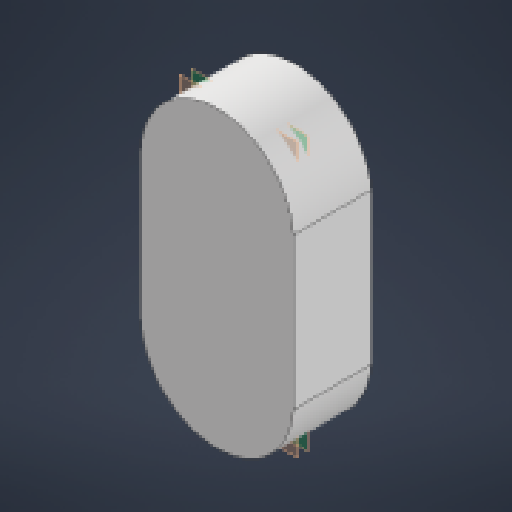
# Autodesk Inventor part: battery_case_top
Saved by Autodesk Inventor 2024 (Build 280153000, 153)
## iProperties
Created: 2026-08-20
Part Number: battery_case_top
Material: Generic
Document SubType Name: Modeling
Designer: schar
Density: 1 g/cm^3
Appearance: Default
Author: schar
Autodesk Inventor part; units mm, degrees
ref_plane "YZ Plane" through (0, 0, 0) normal (1, 0, 0) x (0, 1, 0)
ref_plane "XZ Plane" through (0, 0, 0) normal (0, 1, 0) x (-1, 0, 0)
ref_plane "XY Plane" through (0, 0, 0) normal (0, 0, 1) x (1, 0, 0)
ref_plane "Work Plane1" through (0, 0, 0) normal (0, 0, 1) x (1, 0, 0)
sketch "Sketch1" plane through (0, 0, 0) normal (0, 0, 1) x (1, 0, 0)
  line L0 (115.3806, -128.0116) -> (115.3806, -106.9325) projected
  arc A0 (115.3806, -106.9325) -> (100.4, -107.4721) centre (107.9, -107.4721) ccw projected
  line L1 (100.4, -127.4721) -> (100.4, -107.4721) projected
  arc A1 (100.4, -127.4721) -> (115.3806, -128.0116) centre (107.9, -127.4721) ccw projected
  circle A2 centre (112.8806, -107.5) radius 0.5 projected
  circle A3 centre (102.1806, -116.425) radius 0.5 projected
  circle A4 centre (102.1806, -118.965) radius 0.5 projected
  circle A5 centre (112.8806, -127.5) radius 0.5 projected
  line L2 (118.6109, -126.102) -> (118.6109, -108.8422) projected
  arc A6 (118.3353, -104.9731) -> (97.3428, -105.5521) centre (107.9, -107.4721) ccw projected
  line L3 (97.1697, -109.4876) -> (97.1697, -125.4565) projected
  arc A7 (97.3428, -129.392) -> (118.3353, -129.971) centre (107.9, -127.4721) ccw projected
  arc A8 (98.8697, -116.3059) -> (98.8697, -118.6383) centre (102.1697, -117.4721) ccw projected
  line L4 (98.8697, -116.3059) -> (98.8697, -107.4721) projected
  arc A9 (116.9109, -106.88) -> (98.8697, -107.4721) centre (107.9, -107.4721) ccw projected
  line L5 (116.9109, -106.88) -> (116.9109, -128.0642) projected
  arc A10 (98.8697, -127.4721) -> (116.9109, -128.0642) centre (107.9, -127.4721) ccw projected
  line L6 (98.8697, -127.4721) -> (98.8697, -118.6383) projected
  arc A11 (118.3353, -129.971) -> (118.6109, -126.102) centre (119.6109, -128.1176) ccw projected
  arc A12 (118.6109, -108.8422) -> (118.3353, -104.9731) centre (119.6109, -106.8266) ccw projected
  arc A13 (97.3428, -105.5521) -> (97.1697, -109.4876) centre (96.1697, -107.4721) ccw projected
  arc A14 (97.1697, -125.4565) -> (97.3428, -129.392) centre (96.1697, -127.4721) ccw projected
  circle A15 centre (96.1697, -127.4721) radius 1.5 projected
  circle A16 centre (119.6109, -128.1176) radius 1.5 projected
  circle A17 centre (96.1697, -107.4721) radius 1.5 projected
  circle A18 centre (119.6109, -106.8266) radius 1.5 projected
  point P0 (0, 0)
extrude "Extrusion1" add sketch "Sketch1" along normal blind 3 contours A1 L1 A0 L0 | A2 | A3 | A4 | A5
ref_plane "Work Plane2" through (0, 0, -1.51) normal (0, 0, -1) x (-1, 0, 0)
ref_plane "Work Plane3" through (97.1697, -138.2024, -7.9168) normal (0, 0, 1) x (1, 0, 0)
body "Solid1"
